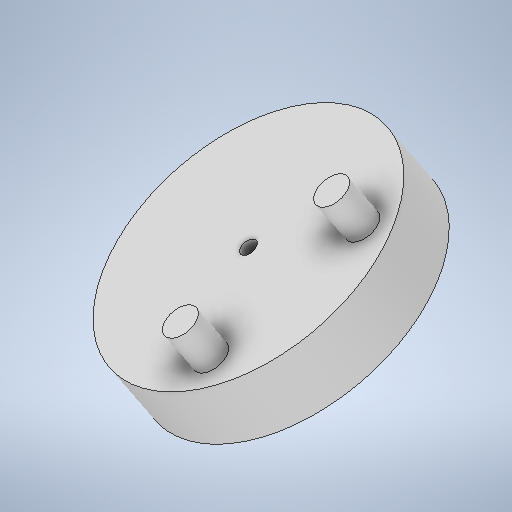
# Autodesk Inventor part: Kupplungsscheibe_v2
Saved by Autodesk Inventor 2025 (Build 290162000, 162)
## iProperties
Created: 2026-06-23
Part Number: Kupplungsscheibe_v2
Material: Generisch
Document SubType Name: Modeling
Designer: GemmiDad-GBSE
Density: 1 g/cm^3
Appearance: Vorgabe
Author: GemmiDad-GBSE
Autodesk Inventor part; units mm, degrees
ref_plane "YZ Plane" through (0, 0, 0) normal (1, 0, 0) x (0, 1, 0)
ref_plane "XZ Plane" through (0, 0, 0) normal (0, 1, 0) x (-1, 0, 0)
sketch "Skizze1" plane through (0, 0, 0) normal (0, 0, 1) x (1, 0, 0)
  circle A0 centre (0, 0) radius 26
  constraints: 1 centre point
extrude "Extrusion1" add sketch "Skizze1" along normal blind 12
ref_plane "Arbeitsebene1" through (0, 0, 12) normal (0, 0, 1) x (1, 0, 0)
sketch "Skizze2" plane through (0, 0, 0) normal (0, 0, 1) x (1, 0, 0)
  circle A0 centre (0, 0) radius 1.5
  constraints: 1 centre point
extrude "Extrusion2" cut sketch "Skizze2" along normal blind 13
sketch "Skizze3" plane through (0, 0, 12) normal (0, 0, 1) x (1, 0, 0)
  circle A0 centre (20, 0) radius 3
  constraints: 1 centre point
extrude "Extrusion3" add sketch "Skizze3" along normal blind 8 separate body
sketch "Skizze4" plane through (0, 0, 12) normal (0, 0, 1) x (1, 0, 0)
  circle A0 centre (0, 20) radius 3
  constraints: 1 centre point
extrude "Extrusion4" add sketch "Skizze4" along normal blind 8 separate body
sketch "Skizze5" plane through (0, 0, 0) normal (0, 0, 1) x (1, 0, 0)
  circle A0 centre (20, 0) radius 2
  constraints: 1 centre point
extrude "Extrusion5" cut sketch "Skizze5" along normal blind 12 bodies 1
sketch "Skizze6" plane through (0, 0, 0) normal (0, 0, 1) x (1, 0, 0)
  circle A0 centre (9.1924, 9.1924) radius 5
  circle A1 centre (-9.1924, 9.1924) radius 5
  circle A2 centre (-9.1924, -9.1924) radius 5
  circle A3 centre (9.1924, -9.1924) radius 5
  constraints: 4 centre point
extrude "Extrusion6" cut sketch "Skizze6" along normal blind 8 bodies 1
